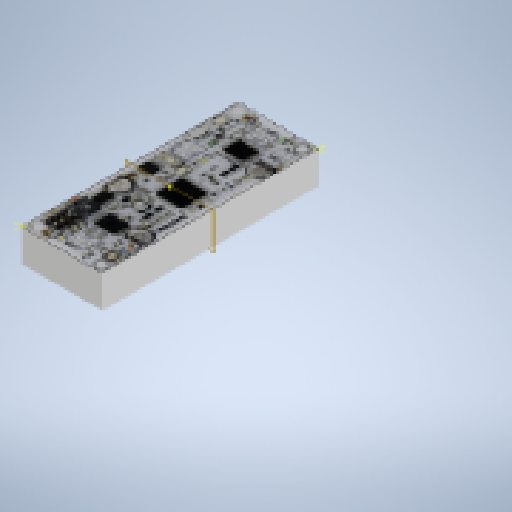
# Autodesk Inventor part: board
Saved by Autodesk Inventor 2024 (Build 280153000, 153)
## iProperties
Created: 2023-10-20
Part Number: board
Material: Generic
Document SubType Name: Modeling
Designer: kdcao
Density: 1 g/cm^3
Appearance: Default
Author: kdcao
Autodesk Inventor part; units mm, degrees
ref_plane "YZ Plane" through (0, 0, 0) normal (1, 0, 0) x (0, 1, 0)
ref_plane "XZ Plane" through (0, 0, 0) normal (0, 1, 0) x (-1, 0, 0)
ref_plane "XY Plane" through (0, 0, 0) normal (0, 0, 1) x (1, 0, 0)
sketch "Sketch1" plane through (0, 0, 0) normal (0, 1, 0) x (-1, 0, 0)
  line L0 (-15, 40) -> (15, 40)
  line L1 (15, 40) -> (15, -40)
  line L2 (15, -40) -> (-15, -40)
  line L3 (-15, -40) -> (-15, 40)
  line L4 (-15, 40) -> (15, -40) construction
  line L5 (15, 40) -> (-15, -40) construction
  point P0 (0, 0)
  dimension "d0" = 80
  dimension "d1" = 30
  constraints: 12 end point, 2 midpoint, 2 parallel, 1 horizontal, 1 perpendicular
  measures "d0" distance of L0.end L1.end
  measures "d1" distance of L0.start L0.end
extrude "Extrusion1" add sketch "Sketch1" along normal blind 12
sketch "Sketch2" plane through (0, 12, 0) normal (0, 1, 0) x (1, 0, 0)
  line L0 (15, 40) -> (14.4693, -40.195) construction
  line L1 (14.4693, -40.195) -> (-15, -40) construction
  line L2 (-15, -40) -> (-14.4693, 40.195) construction
  line L3 (-14.4693, 40.195) -> (15, 40) construction
  point P0 (0, 0)
  constraints: 2 coincident, 2 other
ref_plane "Work Plane1" through (-15, 0, 0) normal (0, 0, 1) x (1, 0, 0)
body "Solid1"
